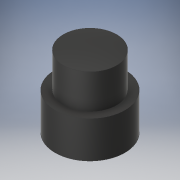
# Autodesk Inventor part: GUI button
Saved by Autodesk Inventor 2018 (Build 220112000, 112)
## iProperties
Created: 2013-10-28
Part Number: GUI button
Material: Nylon 6/6
Document SubType Name: Modeling
Designer: Gabriel Smolnycki
Mass: 0.430568 g
Surface Area: 3.42332 cm^2
Volume: 0.381033 cm^3
Density: 1.13 g/cm^3
Appearance: Smooth - Black
Sending System: SolidWorks 2017
Last Author: Gabriel Smolnycki
Last Saved: 2017-09-14
Author: Gabriel Smolnycki
Autodesk Inventor part; units mm, degrees
ref_plane "YZ Plane" through (0, 0, 0) normal (1, 0, 0) x (0, 1, 0)
ref_plane "XZ Plane" through (0, 0, 0) normal (0, 1, 0) x (-1, 0, 0)
ref_plane "XY Plane" through (0, 0, 0) normal (0, 0, 1) x (1, 0, 0)
sketch "Sketch1" plane through (0, 0, 0) normal (0, 0, 1) x (1, 0, 0)
  line L0 (-1.75, 0) -> (-4.25, 0)
  arc A0 (0, 9) -> (-3.25, 8.7342) centre (0, -11) ccw
  line L1 (-1.75, 0) -> (-1.75, 2)
  line L2 (-3.25, 4.5) -> (-4.25, 4.5)
  line L3 (-3.25, 8.7342) -> (-3.25, 4.5)
  line L4 (0, 2) -> (-1.75, 2)
  line L5 (-4.25, 4.5) -> (-4.25, 0)
  line L6 (0, 9) -> (0, 2)
  line L7 (0, 2) -> (0, -8)
  constraints: 16 end point, 5 vertical, 3 horizontal, 2 point on circle, 1 centre point
revolve "Revolution1" add sketch "Sketch1" angle 360 about axis through (0, 2, 0) along (0, -1, 0)
body "Solid3"
